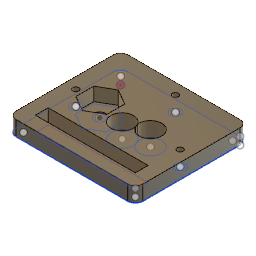
TeamScheire_Sara v22 (Autodesk Fusion 360 design; units mm, degrees)
Autodesk Fusion 360 part; units mm, degrees
sketch "Sketch1" plane through (0, 0, 0) normal (0, 1, 0) x (1, 0, 0)
  line L0 (65, -55.2) -> (0, -55.2)
  line L1 (70, -65.2) -> (-5, -65.2) construction
  line L2 (-10, -60.2) -> (-10, 5) construction
  line L3 (-5, 10) -> (70, 10) construction
  line L4 (75, 5) -> (75, -60.2) construction
  line L5 (0, -55.2) -> (65, -55.2) construction
  line L6 (65, -55.2) -> (65, -48.596) construction
  line L7 (65, -48.596) -> (0, -48.596) construction
  line L8 (0, -48.596) -> (0, -55.2) construction
  line L9 (-1, -56.2) -> (66, -56.2) construction
  line L10 (66, -56.2) -> (66, -47.596) construction
  line L11 (66, -47.596) -> (-1, -47.596) construction
  line L12 (-1, -47.596) -> (-1, -56.2) construction
  line L13 (22.4924, -32.1613) -> (22.4924, -20.1613)
  line L14 (22.4924, -20.1613) -> (12.1001, -14.1613)
  line L15 (12.1001, -14.1613) -> (1.7078, -20.1613)
  line L16 (1.7078, -20.1613) -> (1.7078, -32.1613)
  line L17 (1.7078, -32.1613) -> (12.1001, -38.1613)
  line L18 (12.1001, -38.1613) -> (22.4924, -32.1613)
  circle A0 centre (32, -31) radius 7.5
  circle A1 centre (46, -26) radius 7.5
  circle A2 centre (-2.5, -27.6) radius 2
  circle A3 centre (67.5, -27.6) radius 2
  line L19 (-5, 10) -> (70, 10)
  line L20 (75, 5) -> (75, -60.2)
  line L21 (70, -65.2) -> (-5, -65.2)
  line L22 (-10, -60.2) -> (-10, 5)
  line L23 (66, -56.2) -> (-1, -56.2)
  line L24 (-1, -56.2) -> (-1, -47.596)
  line L25 (-1, -47.596) -> (66, -47.596)
  line L26 (66, -47.596) -> (66, -56.2)
  arc A4 (-5, 10) -> (-10, 5) centre (-5, 5) ccw
  arc A5 (75, 5) -> (70, 10) centre (70, 5) ccw
  arc A6 (70, -65.2) -> (75, -60.2) centre (70, -60.2) ccw
  arc A7 (70, -65.2) -> (75, -60.2) centre (70, -60.2) ccw
  arc A8 (-5, 10) -> (-10, 5) centre (-5, 5) ccw
  arc A9 (-10, -60.2) -> (-5, -65.2) centre (-5, -60.2) ccw construction
  arc A10 (-10, -60.2) -> (-5, -65.2) centre (-5, -60.2) ccw
  circle A11 centre (-2.5, -27.6) radius 2
  circle A12 centre (34.2445, 2.5) radius 2
  circle A13 centre (12.1001, -26.1613) radius 3.5
  circle A14 centre (-2.5, -27.6) radius 3.5
  circle A15 centre (34.2445, 2.5) radius 3.5
  circle A16 centre (67.5, -27.6) radius 3.5
  point P0 (12.1001, -26.1613)
  dimension "d2" = 55.2
  dimension "d12" = 6.604
  dimension "d13" = 1
  dimension "d14" = 12
  dimension "d17" = 15
  dimension "d20" = 15
  dimension "d23" = 4
  dimension "d24" = 4
  dimension "d27" = 27.6
  dimension "d28" = 27.6
  dimension "d31" = 5
  dimension "d33" = 5
  dimension "d34" = 5
  dimension "d35" = 5
  dimension "d36" = 5
  dimension "d45" = 4
  dimension "d46" = 4
  dimension "d47" = 34.2445
  dimension "d49" = 7.5
  dimension "d55" = 7
  dimension "d61" = 7
  dimension "d62" = 7
  dimension "d63" = 7
  constraint horizontal L0
  constraint horizontal L5
  constraint vertical L6
  constraint horizontal L7
  constraint vertical L8
  constraint horizontal L19
  constraint vertical L20
  constraint horizontal L21
  constraint vertical L22
  constraint horizontal L23
  constraint vertical L24
  constraint horizontal L25
  constraint vertical L26
  constraint parallel L0 L1
  constraint tangent L3 A4
  constraint tangent L22 A4
  constraint tangent L19 A5
  constraint tangent L20 A5
  constraint tangent L4 A6
  constraint tangent L21 A6
  constraint tangent L1 A7
  constraint tangent L20 A7
  constraint equal A6 A7
  constraint tangent L2 A8
  constraint tangent L19 A8
  constraint tangent L1 A9
  constraint tangent L2 A9
  constraint tangent L21 A10
  constraint tangent L22 A10
  constraint equal A9 A10
  constraint parallel L2 L16
  constraint coincident P0 A13.centre
  constraint concentric A11 A14
  constraint concentric A12 A15
  constraint concentric A3 A16
  measures "d2" distance of origin L0.end
  measures "d12" distance of L0.end L7.end
  measures "d14" distance of L13.start P0
  measures "d17" diameter of A0
  measures "d20" diameter of A1
  measures "d23" diameter of A2
  measures "d24" diameter of A3
  measures "d27" distance of L0 A3.centre
  measures "d28" distance of L0 A2.centre
  measures "d31" radius of A4
  measures "d33" radius of A5
  measures "d34" radius of A6
  measures "d35" radius of A8
  measures "d36" radius of A9
  measures "d45" diameter of A11
  measures "d46" diameter of A12
  measures "d47" distance of L8 A12.centre
  measures "d49" distance of L19 A12.centre
  measures "d55" diameter of A13
  measures "d61" diameter of A14
  measures "d62" diameter of A15
  measures "d63" diameter of A16
extrude "Extrude1" add sketch "Sketch1" along normal blind 10 contours L13 L14 L15 L16 L17 L18 | A0 A1 | A0 A1 | A0 A1 | A2 A11 | A3 | L19 L20 L21 L22 A4 A5 A6 A7 A8 A10 | A12 | A13 | A14 | A15 | A16
extrude "Extrude2" cut sketch "Sketch1" along normal blind 10 contours A0 A1 picked at (29.7352, -32.1613)
extrude "Extrude3" cut sketch "Sketch1" along normal blind 10 contours A0 A1 picked at (48.3075, -24.9453)
extrude "Extrude4" cut sketch "Sketch1" along normal blind 10 contours A3
extrude "Extrude5" cut sketch "Sketch1" along normal blind 10 contours A2 A11
extrude "Extrude6" cut sketch "Sketch1" along normal blind 10 contours A12
ref_plane "WorkPlane1" through (32.5, 10, 27.6) normal (0, 1, 0) x (1, 0, 0)
sketch "Sketch2" plane through (32.5, 10, 27.6) normal (0, 1, 0) x (1, 0, 0)
  line L0 (-30.7922, -4.1613) -> (-20.3999, -10.1613)
  line L1 (-20.3999, -10.1613) -> (-10.0076, -4.1613)
  line L2 (-10.0076, -4.1613) -> (-10.0076, 7.8387)
  line L3 (-10.0076, 7.8387) -> (-20.3999, 13.8387)
  line L4 (-20.3999, 13.8387) -> (-30.7922, 7.8387)
  line L5 (-30.7922, 7.8387) -> (-30.7922, -4.1613)
extrude "Extrude7" cut sketch "Sketch2" against normal blind 9
extrude "Extrude8" cut sketch "Sketch1" along normal blind 10 contours A13
sketch "Sketch3" plane through (0, 10, 0) normal (0, 1, 0) x (-1, 0, 0)
  line L0 (-12.1001, 37.7613) -> (-1.7078, 31.7613)
  line L1 (-1.7078, 31.7613) -> (-1.7078, 19.7613)
  line L2 (-1.7078, 19.7613) -> (-12.1001, 13.7613)
  line L3 (-12.1001, 13.7613) -> (-22.4924, 19.7613)
  line L4 (-22.4924, 19.7613) -> (-22.4924, 31.7613)
  line L5 (-22.4924, 31.7613) -> (-12.1001, 37.7613)
  circle A0 centre (-34.2445, -2.5) radius 2
  circle A1 centre (2.5, 27.6) radius 2
  circle A2 centre (-67.5, 27.6) radius 2
  arc A3 (5, -10) -> (10, -5) centre (5, -5) ccw
  line L6 (10, -5) -> (10, 60.2)
  arc A4 (10, 60.2) -> (5, 65.2) centre (5, 60.2) ccw
  line L7 (5, 65.2) -> (-70, 65.2)
  arc A5 (-70, 65.2) -> (-75, 60.2) centre (-70, 60.2) ccw
  line L8 (-75, 60.2) -> (-75, -5)
  arc A6 (-75, -5) -> (-70, -10) centre (-70, -5) ccw
  line L9 (-70, -10) -> (5, -10)
  line L10 (1, 47.596) -> (-66, 47.596)
  line L11 (-66, 47.596) -> (-66, 56.2)
  line L12 (-66, 56.2) -> (1, 56.2)
  line L13 (1, 56.2) -> (1, 47.596)
  arc A7 (-39.3363, 29.4417) -> (-38.6637, 27.5583) centre (-46, 26) ccw
  arc A8 (-38.6637, 27.5583) -> (-39.3363, 29.4417) centre (-32, 31) ccw
ref_plane "WorkPlane2" through (32.5, 14, 27.6) normal (0, 1, 0) x (-1, 0, 0)
ref_plane "WorkPlane3" through (32.5, 15, 27.6) normal (0, 1, 0) x (-1, 0, 0)
ref_plane "WorkPlane4" through (32.5, 10, 27.6) normal (0, 1, 0) x (-1, 0, 0)
extrude "Extrude9" cut sketch "Sketch1" along normal blind 2 contours A14
extrude "Extrude10" cut sketch "Sketch1" along normal blind 2 contours A16
extrude "Extrude11" cut sketch "Sketch1" along normal blind 2 contours A15
